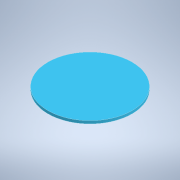
# Autodesk Inventor part: pat
Saved by Autodesk Inventor 2022 (Build 260153000, 153)
## iProperties
Created: 2022-02-27
Part Number: pat
Material: PET Plastic
Document SubType Name: Modeling
Designer: Oana
Density: 1.541 g/cm^3
Appearance: Turquoise
Author: Oana
Autodesk Inventor part; units mm, degrees
ref_plane "YZ Plane" through (0, 0, 0) normal (1, 0, 0) x (0, 1, 0)
ref_plane "XZ Plane" through (0, 0, 0) normal (0, 1, 0) x (-1, 0, 0)
ref_plane "XY Plane" through (0, 0, 0) normal (0, 0, 1) x (1, 0, 0)
sketch "Sketch1" plane through (0, 0, 0) normal (0, 1, 0) x (-1, 0, 0)
  circle A0 centre (0, 0) radius 60
  dimension "d0" = 120
  constraints: 1 centre point, 1 coincident
  measures "d0" diameter of A0
extrude "Extrusion1" add sketch "Sketch1" along normal blind 4
sketch "Sketch2" plane through (0, 0, 0) normal (0, -1, 0) x (1, 0, 0)
  point P0 (0, 0)
sketch "Sketch4" plane through (0, 0, 0) normal (0, -1, 0) x (1, 0, 0)
  circle A0 centre (0, 0) radius 5.5
  dimension "d7" = 11
  constraints: 1 centre point, 1 coincident
  measures "d7" diameter of A0
extrude "Extrusion3" add sketch "Sketch4" along normal blind 5
sketch "Sketch5" plane through (0, 0, 0) normal (0, -1, 0) x (1, 0, 0)
  point P0 (0, 0)
sketch "Sketch8" plane through (0, -5, 0) normal (0, -1, 0) x (1, 0, 0)
  line L0 (3.9692, 4.8706) -> (31.1403, 4.8706)
  line L1 (31.1403, 4.8706) -> (31.1403, -5.1294)
  line L2 (31.1403, -5.1294) -> (3.9692, -5.1294)
  line L3 (3.9692, -5.1294) -> (3.9692, 4.8706)
  point P0 (0, 0)
  dimension "d15" = 10
  constraints: 8 end point, 2 parallel, 1 horizontal, 1 perpendicular
  measures "d15" distance of L2.end L0.start
extrude "Extrusion5" cut sketch "Sketch8" against normal blind 1
equation "\"d0\" = diamteru"
equation "\"d1\" = grosime"
equation "\"diamteru\" = 120"
equation "\"grosime\" = 4"
body "Solid1"
